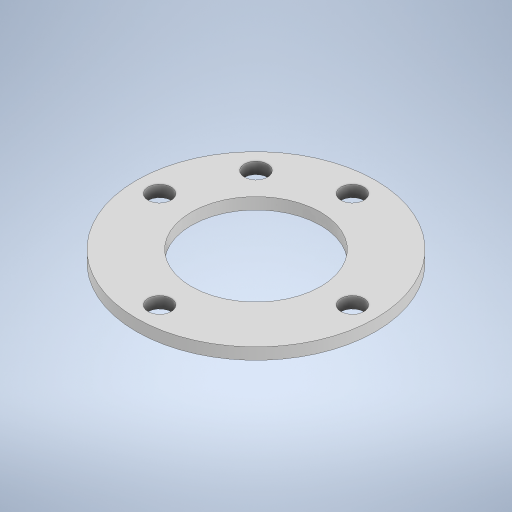
# Autodesk Inventor part: robotiq_ur5_flange_adapter_flattener
Saved by Autodesk Inventor 2023 (Build 270158000, 158)
## iProperties
Created: 2022-06-03
Part Number: robotiq_ur5_flange_adapter_flattener
Material: Generic
Document SubType Name: Modeling
Designer: alt
Density: 1 g/cm^3
Appearance: Default
Author: alt
Autodesk Inventor part; units mm, degrees
ref_plane "YZ Plane" through (0, 0, 0) normal (1, 0, 0) x (0, 1, 0)
ref_plane "XZ Plane" through (0, 0, 0) normal (0, 1, 0) x (-1, 0, 0)
ref_plane "XY Plane" through (0, 0, 0) normal (0, 0, 1) x (1, 0, 0)
sketch "Sketch2" plane through (0, 0, 0) normal (0, 1, 0) x (-1, 0, 0)
  circle A0 centre (0, 0) radius 16.75
  circle A1 centre (0, 0) radius 25
  circle A2 centre (0, 0) radius 31
  circle A3 centre (25, 0) radius 3
  circle A4 centre (0, 25) radius 3
  circle A5 centre (0, -25) radius 3
  circle A6 centre (-25, 0) radius 3
  circle A7 centre (17.6777, -17.6777) radius 3
  line L0 (0, 0) -> (25, 0)
  line L1 (0, 0) -> (17.6777, -17.6777)
  dimension "d0" = 33.5
  dimension "d1" = 50
  dimension "d2" = 62
  dimension "d3" = 6
  dimension "d4" = 6
  dimension "d5" = 45
  constraints: 8 centre point, 5 point on circle, 4 end point, 3 coincident, 3 equal radius, 1 horizontal
  measures "d0" diameter of A0
  measures "d1" diameter of A1
  measures "d2" diameter of A2
  measures "d3" diameter of A3
  measures "d4" diameter of A7
  measures "d5" angle of L0 L1
extrude "Extrusion1" add sketch "Sketch2" along normal blind 3 contours L0 A3 A1 A7 L1 A0 | A0 L1 A7 A1 A5 A6 A4 A3 L0 | A2
body "Solid1"
